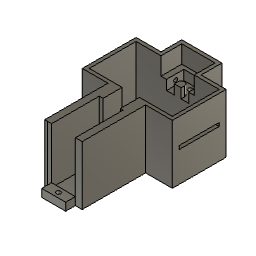
table_base (Autodesk Fusion 360 design; units mm, degrees)
Autodesk Fusion 360 part; units mm, degrees
sketch "Sketch1" plane through (0, 0, 0) normal (0, 0, 1) x (1, 0, 0)
  line L0 (76.2, 25.4) -> (0, 25.4)
  line L1 (48.6484, -35) -> (48.6484, -85)
  line L2 (26.6484, -76) -> (26.6484, -85)
  line L3 (48.6484, -76) -> (48.6484, -35)
  line L4 (26.6484, -35) -> (26.6484, -76)
  line L5 (30.1, -17.526) -> (30.1, -34.9936)
  line L6 (46.1, -34.9936) -> (46.1, -17.526)
  circle A0 centre (37.6484, -83.3194) radius 2.05
  line L7 (37.6484, -81.2694) -> (37.6484, -80.5) construction
  line L8 (48.6484, -76.0942) -> (48.6484, -35)
  line L9 (26.6484, -75.9063) -> (26.6484, -35)
  line L10 (46.1, -17.526) -> (46.1, -34.9936)
  line L11 (30.1, -34.9936) -> (26.6484, -34.9936)
  line L12 (30.1, -17.526) -> (30.1, -34.9936)
  line L13 (0, 25.4) -> (76.2, 25.4)
  line L14 (79.375, 28.575) -> (-3.175, 28.575)
  line L15 (30.1, -17.526) -> (30.1, -34.9936)
  line L16 (30.1, -34.9936) -> (26.6484, -34.9936)
  line L17 (26.6484, -34.9936) -> (26.6484, -75.9063)
  line L18 (46.1, -17.526) -> (46.1, -34.9936)
  line L19 (46.1, -34.9936) -> (48.6484, -34.9936)
  line L20 (48.6484, -34.9936) -> (48.6484, -76.0942)
  line L21 (46.1, -34.9936) -> (48.6484, -34.9936)
  line L22 (26.6484, -75.9063) -> (26.6484, -78.7257)
  line L23 (26.6484, -78.7257) -> (48.6484, -78.9136)
  line L24 (48.6484, -85) -> (48.6484, -78.9136)
  line L25 (48.6484, -76.0942) -> (48.6484, -76)
  line L26 (26.6484, -85) -> (26.6484, -78.7257)
  line L27 (26.6484, -75.9063) -> (26.6484, -35)
  line L28 (52.3234, -78.9136) -> (48.6484, -78.9136)
  line L29 (22.9734, -78.7257) -> (26.6484, -78.7257)
  line L30 (26.6484, -85) -> (26.6484, -87.8194)
  line L31 (48.6484, -85) -> (48.6484, -87.8194)
  line L32 (48.6484, -87.8194) -> (26.6484, -87.8194)
  line L33 (20.32, -78.74) -> (20.32, -66.04)
  line L34 (20.32, -66.04) -> (20.32, -20.701)
  line L35 (22.9734, -78.7257) -> (20.32, -78.74)
  line L36 (52.3234, -78.9136) -> (54.8634, -78.9136)
  line L37 (54.8634, -78.9136) -> (54.8634, -20.701)
  line L38 (-3.1761, -11.938) -> (-3.175, -11.938)
  line L39 (76.1981, -17.526) -> (46.1, -17.526)
  line L40 (30.1, -17.526) -> (0, -17.526)
  line L41 (-3.173, -20.701) -> (20.32, -20.701)
  line L42 (54.8634, -20.701) -> (79.3731, -20.701)
  line L43 (76.2, 25.4) -> (76.1981, -17.526)
  line L44 (79.375, 28.575) -> (79.3731, -20.701)
  line L45 (0, 25.4) -> (0, -17.526)
  line L46 (-3.175, 28.575) -> (-3.173, -20.701)
  point P0 (38.1, 0)
  point P1 (38.1, -15)
  point P2 (37.6484, 0)
  dimension "d2" = 25.4
  dimension "d5" = 9
  dimension "d6" = 41
  dimension "d9" = 16
  dimension "d12" = 4.1
  dimension "d47" = 2.8194
  dimension "d48" = 2.8194
  dimension "d50" = 2.8194
  dimension "d51" = 2.8194
  dimension "d53" = 2.54
  constraint horizontal L0
  constraint vertical L1
  constraint vertical L26
  constraint vertical L24
  constraint vertical L2
  constraint vertical L3
  constraint vertical L4
  constraint parallel L5 L6
  constraint vertical L8
  constraint vertical L9
  constraint horizontal L21
  constraint vertical L10
  constraint horizontal L11
  constraint vertical L12
  constraint horizontal L13
  constraint horizontal L14
  constraint vertical L15
  constraint horizontal L16
  constraint vertical L17
  constraint vertical L18
  constraint horizontal L19
  constraint vertical L20
  constraint collinear L24 L25
  constraint collinear L26 L27
  constraint coincident A0 L7.start
  constraint perpendicular L29 L33
  constraint coincident L5.start L39
  constraint collinear L39 L40
  constraint collinear L41 L42
  constraint vertical L45
  measures "d2" distance of origin L0.end
  measures "d5" distance of L2.end L2.start
  measures "d6" distance of L2.start L4.start
  measures "d9" distance of L5.end L6.start
  measures "d12" diameter of A0
  measures "d47" distance of L9.start L22.end
  measures "d48" distance of L8.start L23.end
  measures "d50" distance of L2.end L30.end
  measures "d51" distance of L1.end L31.end
  measures "d53" distance of L28.start L36.end
extrude "Extrude7" add sketch "Sketch1" against normal blind 3.175 makes body 1
extrude "Extrude8" add sketch "Sketch1" along normal blind 50.8 contours L0 L1 L2 L3 L4 L5 L6 L8 L9 L10 L11 L12 L13 L14 L15 L16 L17 L18 L19 L20 L21 L22 L25 L27 L28 L29 L33 L34 L35 L36 L37 L39 L40 L41 L42 L43 L44 L45 L46 bodies 1
extrude "Extrude10" add sketch "Sketch1" along normal blind 4 contours L1 L2 L23 L24 L26 L30 L31 L32 bodies 1
sketch "Sketch3" plane through (0, 28.575, 0) normal (0, 1, 0) x (-1, 0, 0)
  line L0 (-79.375, 50.8) -> (-79.375, -3.175)
  line L1 (-79.375, -3.175) -> (3.175, -3.175)
  line L2 (3.175, -3.175) -> (3.175, 50.8)
  line L3 (3.175, 50.8) -> (-79.375, 50.8)
  line L4 (-53.34, 20.32) -> (-22.86, 20.32)
  line L5 (-22.86, 20.32) -> (-22.86, 34.6202)
  line L6 (-22.86, 34.6202) -> (-53.34, 34.6202)
  line L7 (-53.34, 34.6202) -> (-53.34, 20.32)
  dimension "d87" = 30.48
  dimension "d88" = 14.3002
  constraint horizontal L4
  constraint vertical L5
  constraint horizontal L6
  constraint vertical L7
  measures "d87" distance of L4.start L4.end
  measures "d88" distance of L4.start L6.end
extrude "Extrude11" add sketch "Sketch3" along normal blind 15.875 separate body contours L4 L5 L6 L7 makes body 2
sketch "Sketch4" plane through (0, 0, 34.6202) normal (0, 0, 1) x (-1, 0, 0)
  line L0 (-22.86, -28.575) -> (-53.34, -28.575)
  line L1 (-53.34, -28.575) -> (-53.34, -44.45)
  line L2 (-53.34, -44.45) -> (-22.86, -44.45)
  line L3 (-22.86, -44.45) -> (-22.86, -28.575)
  line L4 (-48.26, -28.575) -> (-27.94, -28.575)
  line L5 (-27.94, -28.575) -> (-27.94, -41.275)
  line L6 (-27.94, -41.275) -> (-48.26, -41.275)
  line L7 (-48.26, -41.275) -> (-48.26, -28.575)
  circle A0 centre (-38.1, -28.575) radius 3.175
  dimension "d91" = 20.32
  dimension "d92" = 12.7
  dimension "d93" = 5.08
  dimension "d94" = 6.35
  constraint horizontal L4
  constraint vertical L5
  constraint horizontal L6
  constraint vertical L7
  constraint coincident L0 L4.start
  constraint midpoint L4 A0.centre
  measures "d91" distance of L4.start L4.end
  measures "d92" distance of L4.start L6.end
  measures "d93" distance of L3 L5
  measures "d94" diameter of A0
extrude "Extrude12" cut sketch "Sketch4" against normal blind 8.89 contours L0 L4 L5 L6 L7 A0 bodies 2
sketch "Sketch5" plane through (22.86, 0, 0) normal (-1, 0, 0) x (0, -1, 0)
  line L0 (-28.575, 20.32) -> (-28.575, 34.6202)
  line L1 (-28.575, 34.6202) -> (-44.45, 34.6202)
  line L2 (-44.45, 34.6202) -> (-44.45, 20.32)
  line L3 (-44.45, 20.32) -> (-28.575, 20.32)
  circle A0 centre (-33.7311, 29.984) radius 1.778
  dimension "d97" = 3.556
  measures "d97" diameter of A0
extrude "Extrude13" cut sketch "Sketch5" against normal blind 48.26 contours A0 bodies 2
extrude "Extrude14" add 1 faces at (43.18, 44.45, 25.0867) along direction (0, 1, 0) blind 3.175 on bodies 2 bodies 2
extrude "Extrude15" add 1 faces at (22.86, 43.56, 28.1334) along direction (-1, 0, 0) blind 3.175 on bodies 2 bodies 1 2
extrude "Extrude16" add 1 faces at (53.34, 43.56, 28.1334) along direction (1, 0, 0) blind 3.175 on bodies 1 bodies 1
extrude "Extrude17" add 1 faces at (22.4367, 39.1583, 34.6202) along direction (0, 0, 1) up to surface (16.1798 mm away) on bodies 1 bodies 1
sketch "Sketch6" plane through (0, 0, 50.8) normal (0, 0, 1) x (-1, 0, 0)
  line L0 (-48.26, -28.575) -> (-27.94, -28.575)
  line L1 (-27.94, -28.575) -> (-27.94, -41.275)
  line L2 (-27.94, -41.275) -> (-48.26, -41.275)
  line L3 (-48.26, -41.275) -> (-48.26, -28.575)
  line L4 (-56.515, -28.575) -> (-56.515, -47.625)
  line L5 (-56.515, -47.625) -> (-19.685, -47.625)
  line L6 (-19.685, -47.625) -> (-19.685, -28.575)
  line L7 (-19.685, -28.575) -> (3.175, -28.575)
  line L8 (3.175, -28.575) -> (3.173, 20.701)
  line L9 (3.173, 20.701) -> (-20.32, 20.701)
  line L10 (-20.32, 20.701) -> (-20.32, 78.74)
  line L11 (-20.32, 78.74) -> (-22.9734, 78.7257)
  line L12 (-22.9734, 78.7257) -> (-26.6484, 78.7257)
  line L13 (-26.6484, 78.7257) -> (-26.6484, 34.9936)
  line L14 (-26.6484, 34.9936) -> (-30.1, 34.9936)
  line L15 (-30.1, 34.9936) -> (-30.1, 17.526)
  line L16 (-30.1, 17.526) -> (0, 17.526)
  line L17 (0, 17.526) -> (0, -25.4)
  line L18 (0, -25.4) -> (-76.2, -25.4)
  line L19 (-76.2, -25.4) -> (-76.1981, 17.526)
  line L20 (-76.1981, 17.526) -> (-46.1, 17.526)
  line L21 (-46.1, 17.526) -> (-46.1, 34.9936)
  line L22 (-46.1, 34.9936) -> (-48.6484, 34.9936)
  line L23 (-48.6484, 34.9936) -> (-48.6484, 78.9136)
  line L24 (-48.6484, 78.9136) -> (-54.8634, 78.9136)
  line L25 (-54.8634, 78.9136) -> (-54.8634, 20.701)
  line L26 (-54.8634, 20.701) -> (-79.3731, 20.701)
  line L27 (-79.3731, 20.701) -> (-79.375, -28.575)
  line L28 (-79.375, -28.575) -> (-56.515, -28.575)
  line L29 (-53.34, -28.575) -> (-22.86, -28.575)
  line L30 (-22.86, -28.575) -> (-22.86, -44.45)
  line L31 (-22.86, -44.45) -> (-53.34, -44.45)
  line L32 (-53.34, -44.45) -> (-53.34, -28.575)
  dimension "d108" = 30.48
  dimension "d109" = 15.875
  dimension "d110" = 3.175
  dimension "d111" = 3.175
  constraint horizontal L29
  constraint vertical L30
  constraint horizontal L31
  constraint vertical L32
  measures "d108" distance of L29.start L29.end
  measures "d109" distance of L29.start L31.end
  measures "d110" distance of L4 L32
  measures "d111" distance of L5 L31
extrude "Extrude18" cut sketch "Sketch6" against normal up to surface (16.1798 mm away) contours L1 L2 L3 L29 L30 L31 L32 bodies 1
extrude "Extrude19" add 1 faces at (44.2383, 34.925, 20.32) along direction (0, 0, -1) up to surface (23.495 mm away) thin wall 3.175 inside on bodies 1 bodies 1
extrude "Extrude20" cut 1 faces at (37.0417, 28.575, 45.4067) along direction (0, -1, 0) blind 10.16 on bodies 1 bodies 1
sketch "Sketch7" plane through (0, 0, 25.7302) normal (0, 0, 1) x (-1, 0, 0)
  arc A0 (-41.275, -28.575) -> (-34.925, -28.575) centre (-38.1, -28.575) ccw
  line L0 (-41.275, -28.575) -> (-41.275, -25.4)
  line L1 (-41.275, -25.4) -> (-48.26, -25.4)
  line L2 (-27.94, -25.4) -> (-34.925, -25.4)
  line L3 (-34.925, -25.4) -> (-34.925, -28.575)
  circle A1 centre (-38.1, -36.9824) radius 2.0447
  line L4 (-48.26, -25.4) -> (-48.26, -41.275)
  line L5 (-48.26, -41.275) -> (-27.94, -41.275)
  line L6 (-27.94, -41.275) -> (-27.94, -25.4)
  line L7 (-22.86, -44.45) -> (-53.34, -44.45)
  dimension "d119" = 4.0894
  dimension "d121" = 7.4676
  measures "d119" diameter of A1
  measures "d121" distance of A1.centre L7
extrude "Extrude21" cut sketch "Sketch7" against normal blind 15.24 contours A1 bodies 1
sketch "Sketch8" plane through (79.3739, -0.0031, 0) normal (1, -0.000039, 0) x (0.000039, 1, 0)
  line L0 (-20.6979, 50.8) -> (-20.6979, -3.175)
  line L1 (-20.6979, -3.175) -> (28.5781, -3.175)
  line L2 (28.5781, -3.175) -> (28.5781, 50.8)
  line L3 (28.5781, 50.8) -> (-20.6979, 50.8)
  line L4 (-14.3479, 27.686) -> (22.2281, 27.686)
  line L5 (22.2281, 27.686) -> (22.2281, 24.511)
  line L6 (22.2281, 24.511) -> (-14.3479, 24.511)
  line L7 (-14.3479, 24.511) -> (-14.3479, 27.686)
  dimension "d124" = 27.686
  dimension "d125" = 6.35
  dimension "d126" = 6.35
  dimension "d129" = 3.175
  constraint horizontal L4
  constraint vertical L5
  constraint horizontal L6
  constraint vertical L7
  measures "d124" distance of L1 L6
  measures "d125" distance of L2 L5
  measures "d126" distance of L0 L7
  measures "d129" distance of L4.start L6.end
extrude "Extrude22" cut sketch "Sketch8" along normal mid plane 22.86 contours L4 L5 L6 L7 bodies 1
sketch "Sketch2" plane through (0, 0, 0) normal (0, 0, 1) x (1, 0, 0)
  line L0 (0, 25.4) -> (76.2, 25.4)
  line L1 (76.2, 25.4) -> (76.2, -11.938)
  line L2 (76.2, -11.938) -> (0, -11.938)
  line L3 (0, -11.938) -> (0, 25.4)
  line L4 (0, 25.4) -> (76.2, 25.4)
  line L5 (76.2, 25.4) -> (76.2, -11.938)
  line L6 (76.2, -11.938) -> (0, -11.938)
  line L7 (0, -11.938) -> (0, 25.4)
  line L8 (-3.175, 28.575) -> (79.375, 28.575)
  line L9 (79.375, 28.575) -> (79.375, -15.113)
  line L10 (-3.175, -15.113) -> (-3.175, 28.575)
  line L11 (-3.175, -15.113) -> (-3.175, -20.701)
  line L12 (79.375, -15.113) -> (79.375, -20.701)
  line L13 (79.375, -20.701) -> (-3.175, -20.701)
  line L14 (0, -11.938) -> (0, -17.526)
  line L15 (76.2, -11.938) -> (76.2, -17.526)
  line L16 (76.2, -17.526) -> (0, -17.526)
  line L17 (79.375, -15.113) -> (76.2, -15.113)
  line L18 (0, -15.113) -> (-3.175, -15.113)
  dimension "d67" = 82.55
  dimension "d68" = 43.688
  dimension "d69" = 3.175
  dimension "d70" = 3.175
  dimension "d71" = 5.588
  dimension "d72" = 5.588
  dimension "d73" = 5.588
  dimension "d74" = 5.588
  constraint horizontal L0
  constraint vertical L1
  constraint horizontal L2
  constraint vertical L3
  constraint horizontal L4
  constraint vertical L5
  constraint horizontal L6
  constraint vertical L7
  constraint horizontal L8
  constraint vertical L9
  constraint horizontal L17
  constraint vertical L10
  constraint perpendicular L11 L17
  constraint perpendicular L12 L17
  constraint perpendicular L14 L17
  constraint perpendicular L15 L17
  constraint coincident L15 L17.end
  constraint coincident L14 L18.start
  constraint collinear L17 L18
  measures "d67" distance of L8.start L8.end
  measures "d68" distance of L8.start L10.start
  measures "d69" distance of L0 L8
  measures "d70" distance of L3 L10
  measures "d71" distance of L10.start L11.end
  measures "d72" distance of L9.end L12.end
  measures "d73" distance of L2.end L14.end
  measures "d74" distance of L1.end L15.end
extrude "Extrude1" [suppressed]
extrude "Extrude9" [suppressed]
extrude "Extrude2" [suppressed]
extrude "Extrude4" [suppressed]
extrude "Extrude5" [suppressed]
extrude "Extrude6" [suppressed]
extrude "Extrude3" [suppressed]
